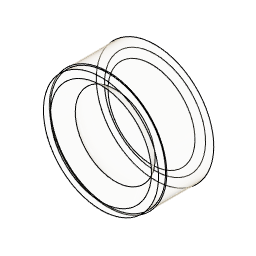
dens-enclosure (Autodesk Fusion 360 archive; units mm, degrees)
design "Focusing Lens"
Autodesk Fusion 360 part; units mm, degrees
sketch "Sketch1" plane through (0, 0, 0) normal (1, 0, 0) x (0, 1, 0)
  line L0 (-1.15, 0) -> (1.15, 0)
  line L1 (0, 2.5) -> (0, -2.5) construction
  line L2 (-1.15, 2.45) -> (-0.85, 2.45)
  line L3 (-0.85, 2.45) -> (-0.85, 2.5)
  line L4 (-0.85, 2.5) -> (1.15, 2.5)
  line L5 (1.15, 2.5) -> (1.15, 2.15)
  line L6 (1.15, -2.15) -> (1.15, -2.5)
  line L7 (1.15, -2.5) -> (-0.85, -2.5)
  line L8 (-0.85, -2.5) -> (-0.85, -2.45)
  line L9 (-0.85, -2.45) -> (-1.15, -2.45)
  line L10 (1.15, 2.15) -> (1, 1.85)
  line L11 (1, -1.85) -> (1.15, -2.15)
  line L12 (1, 1.85) -> (1, -1.85)
  arc A0 (-0.5445, 1.7) -> (-0.5445, -1.7) centre (2.4, 0) ccw
  line L13 (-1.15, 2.45) -> (-1.15, 2.15)
  line L14 (-1.15, -2.45) -> (-1.15, -2.15)
  line L15 (-1.15, 2.15) -> (-0.5445, 1.7)
  line L16 (-0.5445, -1.7) -> (-1.15, -2.15)
  line L17 (-1, 0) -> (1, 0) construction
  dimension "d1" = 2.3
  dimension "d2" = 5
  dimension "d3" = 4.9
  dimension "d4" = 0.3
  dimension "d6" = 4.3
  dimension "d7" = 0.15
  dimension "d8" = 3.7
  dimension "d9" = 3.4
  dimension "d10" = 3.4
  dimension "d11" = 4.3
  dimension "d12" = 2
  constraint horizontal L0
  constraint vertical L1
  constraint symmetric L0 L1.start L1.end
  constraint coincident origin L0
  constraint midpoint origin L0
  constraint midpoint origin L1
  constraint horizontal L2
  constraint perpendicular L2 L3
  constraint perpendicular L3 L4
  constraint perpendicular L4 L5
  constraint vertical L6
  constraint perpendicular L6 L7
  constraint perpendicular L7 L8
  constraint perpendicular L8 L9
  constraint symmetric L0 L2 L9
  constraint collinear L3 L8
  constraint symmetric L0 L4 L7
  constraint coincident L1.start L4
  constraint vertical L0.end L6.start
  constraint collinear L5 L6
  constraint vertical L0.start L9.end
  constraint equal L2 L9
  constraint symmetric L0 L5.end L6.start
  constraint symmetric L0 L11.start L10.end
  constraint symmetric L0 A0.start A0.end
  constraint perpendicular L2 L13
  constraint perpendicular L9 L14
  constraint symmetric L0 L13.end L14.end
  constraint midpoint A0 L17.start
  constraint midpoint L12 L17.end
  measures "d1" distance of L0.start L0.end
  measures "d2" distance of L1.start L1.end
  measures "d3" vertical distance of L2.start L9.end
  measures "d4" distance of L2.start L2.end
  measures "d6" distance of L5.end L6.start
  measures "d7" horizontal distance of L5.end L10.end
  measures "d8" distance of L11.start L10.end
  measures "d9" distance of A0.start A0.end
  measures "d10" radius of A0
  measures "d11" distance of L13.end L14.end
  measures "d12" distance of L17.start L17.end
revolve "Revolve1" add sketch "Sketch1" angle 360 about axis through (0, 1.75, 0) along (0, 1, 0) contours L0 L2 L3 L4 L5 L10 L12 A0 L13 L15

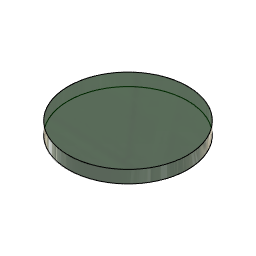
design "UV-IR Cut Filter (BG40)"
Autodesk Fusion 360 part; units mm, degrees
sketch "Sketch1" plane through (0, 0, 0) normal (0, 0, 1) x (1, 0, 0)
  circle A0 centre (0, 0) radius 4.75
  dimension "d1" = 9.5
  constraint coincident A0.centre origin
  measures "d1" diameter of A0
extrude "Extrude1" add sketch "Sketch1" along normal blind 1

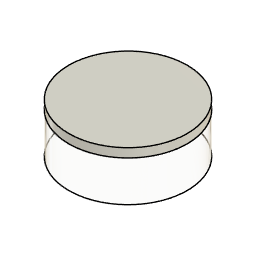
design "Opal Diffuser (6x2.5mm)"
Autodesk Fusion 360 part; units mm, degrees
sketch "Sketch1" plane through (0, 0, 0) normal (0, 0, 1) x (1, 0, 0) in component "Opal Layer"
  circle A0 centre (0, 0) radius 3
  dimension "d1" = 6
  constraint coincident A0.centre origin
  measures "d1" diameter of A0
extrude "Extrude1" add sketch "Sketch1" against normal blind 0.45 makes body 1 in component "Opal Layer"
extrude "Extrude1'" add 1 faces at (-1.1591, 0.5829, -0.45) along direction (0, 0, -1) blind 2.05 separate body on bodies 1 makes body 2 in component "Glass Layer"
component "Opal Layer" placed x (1, 0, 0) y (0, 1, 0) z (0, 0, 1) at (0, 0, 0)
component "Glass Layer" placed x (1, 0, 0) y (0, 1, 0) z (0, 0, 1) at (0, 0, 0)

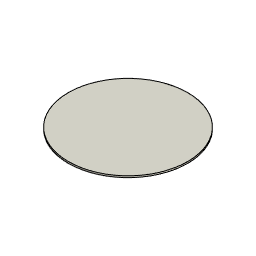
design "Diffuser (0.6in)"
Autodesk Fusion 360 part; units mm, degrees
sketch "Sketch1" plane through (0, 0, 0) normal (0, 0, 1) x (1, 0, 0)
  circle A0 centre (0, 0) radius 7.62
  dimension "d1" = 15.24
  constraint coincident A0.centre origin
  measures "d1" diameter of A0
extrude "Extrude1" add sketch "Sketch1" along normal blind 0.2
